Autodesk Inventor part; units mm, degrees
(part 9 of 18)
  spline S29 degree 3 poles (-103.2775, -7.9462) (-103.2327, -7.9264) (-103.1438, -7.8872) (-103.011, -7.831) (-102.8802, -7.7775) (-102.7099, -7.7106) (-102.5013, -7.6329) (-102.3337, -7.5779) (-102.2514, -7.5508) knots 0 0 0 0 0.13379 0.264806 0.393183 0.519054 0.763783 1 1 1 1
  line L388 (-103.3326, -8.4726) -> (-103.2775, -7.9462)
  spline S30 degree 3 poles (-104.4053, -7.5885) (-104.4187, -7.5896) (-104.4452, -7.5917) (-104.4843, -7.5938) (-104.5221, -7.5949) (-104.5584, -7.595) (-104.5931, -7.594) (-104.6258, -7.5919) (-104.6567, -7.5887) (-104.6856, -7.5845) (-104.7125, -7.5794) (-104.7374, -7.5733) (-104.7601, -7.5664) (-104.7808, -7.5587) (-104.7995, -7.5501) (-104.8165, -7.5405) (-104.8319, -7.5301) (-104.8411, -7.5221) (-104.8455, -7.5181) knots 0 0 0 0 0.088475 0.174424 0.25743 0.337089 0.413015 0.484966 0.552919 0.616878 0.676853 0.732867 0.784956 0.833184 0.87778 0.920162 0.960829 1 1 1 1
  ellipse E254 centre (-100.1455, -8.2742) end of major axis (-105.5768, -7.7059) minor radius 0.0004 (-103.2775, -7.9462) -> (-105.5768, -7.7059) ccw
  line L389 (-105.263, -7.4516) -> (-105.5768, -7.7059)
  line L390 (-105.635, -8.2625) -> (-105.5768, -7.7059)
  spline S31 degree 3 poles (-100.1515, -7.8096) (-100.1089, -7.7854) (-100.0246, -7.7374) (-99.8983, -7.6681) (-99.7738, -7.6016) (-99.6114, -7.5178) (-99.412, -7.4194) (-99.2511, -7.3476) (-99.172, -7.3123) knots 0 0 0 0 0.133763 0.26476 0.393126 0.518994 0.763738 1 1 1 1
  line L391 (-100.1515, -7.9913) -> (-100.1515, -7.8096)
  line L392 (-93.8516, -7.8096) -> (-93.8516, -7.9913)
  spline S32 degree 3 poles (-94.8311, -7.3123) (-94.752, -7.3476) (-94.5911, -7.4194) (-94.3917, -7.5178) (-94.2292, -7.6016) (-94.1047, -7.6681) (-93.9785, -7.7374) (-93.8942, -7.7854) (-93.8516, -7.8096) knots 0 0 0 0 0.236262 0.481006 0.606874 0.73524 0.866237 1 1 1 1
  line L393 (-99.172, -7.3123) -> (-94.8311, -7.3123)
  ellipse E255 centre (-97.0015, -7.7766) end of major axis (-101.9625, -7.7766) minor radius 0.5163 (-94.327, -7.3418) -> (-94.8311, -7.3123) ccw
  ellipse E256 centre (-97.0015, -7.7766) end of major axis (-101.9625, -7.7766) minor radius 0.5163 (-99.172, -7.3123) -> (-99.6761, -7.3418) ccw
  ellipse E257 centre (-97.0015, -8.2739) end of major axis (-91.5405, -8.2739) minor radius 0.5683 (-91.7042, -8.1358) -> (-93.8516, -7.8096) ccw
  ellipse E258 centre (-97.0015, -8.2739) end of major axis (-102.4625, -8.2739) minor radius 0.5683 (-100.1515, -7.8096) -> (-102.2989, -8.1358) ccw
  line L394 (-90.7255, -7.9462) -> (-90.6705, -8.4726)
  spline S33 degree 3 poles (-91.7517, -7.5508) (-91.6694, -7.5779) (-91.5018, -7.6329) (-91.2932, -7.7106) (-91.1229, -7.7775) (-90.9921, -7.831) (-90.8593, -7.8872) (-90.7704, -7.9264) (-90.7255, -7.9462) knots 0 0 0 0 0.236217 0.480946 0.606817 0.735194 0.86621 1 1 1 1
  spline S34 degree 3 poles (-89.158, -7.5179) (-89.1627, -7.5219) (-89.1722, -7.5302) (-89.1885, -7.5409) (-89.2064, -7.5508) (-89.2261, -7.5597) (-89.2476, -7.5676) (-89.2708, -7.5745) (-89.2958, -7.5805) (-89.3224, -7.5854) (-89.3508, -7.5893) (-89.381, -7.5922) (-89.413, -7.5941) (-89.4468, -7.5949) (-89.4823, -7.5947) (-89.5195, -7.5936) (-89.5583, -7.5915) (-89.5847, -7.5893) (-89.5982, -7.5882) knots 0 0 0 0 0.040391 0.082789 0.1275 0.174786 0.22486 0.277901 0.334055 0.393442 0.45616 0.522411 0.592561 0.666584 0.744418 0.825989 0.911213 1 1 1 1
  ellipse E259 centre (-93.8576, -8.2742) end of major axis (-88.4263, -7.7059) minor radius 0.0004 (-88.4263, -7.7059) -> (-90.7255, -7.9462) ccw
  line L395 (-88.7401, -7.4516) -> (-88.4263, -7.7059)
  line L396 (-88.368, -8.2625) -> (-88.4263, -7.7059)
  spline S35 degree 3 poles (-102.8055, -6.0195) (-102.7608, -5.9992) (-102.6724, -5.9592) (-102.5401, -5.9017) (-102.4098, -5.8469) (-102.2402, -5.7784) (-102.0323, -5.6987) (-101.8653, -5.642) (-101.7833, -5.6141) knots 0 0 0 0 0.13379 0.264806 0.393183 0.519054 0.763783 1 1 1 1
  line L397 (-102.9759, -7.8167) -> (-102.8055, -6.0195)
  line L398 (-101.7833, -5.6141) -> (-100.9875, -5.6895)
  ellipse E260 centre (-99.6228, -5.819) end of major axis (-104.5617, -5.3508) minor radius 0.0001 (-104.3919, -5.3669) -> (-104.5617, -5.3508) ccw
  ellipse E261 centre (-99.6228, -5.819) end of major axis (-104.5617, -5.3508) minor radius 0.0001 (-101.7833, -5.6141) -> (-103.1187, -5.4876) ccw
  spline S36 degree 3 poles (-103.1187, -5.4876) (-103.1703, -5.5034) (-103.2713, -5.5344) (-103.4207, -5.5753) (-103.5636, -5.6103) (-103.6994, -5.6388) (-103.8283, -5.6607) (-103.9499, -5.6751) (-104.0464, -5.6809) (-104.118, -5.6805) (-104.1663, -5.6778) (-104.2103, -5.6727) (-104.2501, -5.6655) (-104.2854, -5.6563) (-104.3249, -5.6422) (-104.3662, -5.6193) (-104.4034, -5.5814) (-104.4244, -5.5341) (-104.4269, -5.4805) (-104.4157, -5.4236) (-104.4001, -5.3864) (-104.3919, -5.3669) knots 0 0 0 0 0.104135 0.203976 0.298889 0.388275 0.471711 0.551067 0.624597 0.658204 0.689291 0.717816 0.743784 0.767218 0.788166 0.824633 0.857384 0.888881 0.922221 0.959245 1 1 1 1
  ellipse E262 centre (-99.67, -6.3167) end of major axis (-105.1066, -5.8014) minor radius 0.0001 (-102.8056, -6.0195) -> (-105.1066, -5.8014) ccw
  line L399 (-104.5617, -5.3508) -> (-105.1066, -5.8014)
  ellipse E263 centre (-103.0608, -5.4931) end of major axis (-101.5562, -5.6357) minor radius 0 (-104.3923, -5.3669) -> (-103.2014, -5.4797) ccw
  line L400 (-105.263, -7.4516) -> (-105.1066, -5.8014)
  spline S37 degree 3 poles (-100.1515, -5.896) (-100.1089, -5.8717) (-100.0246, -5.8237) (-99.8983, -5.7543) (-99.7738, -5.6878) (-99.6114, -5.6039) (-99.412, -5.5054) (-99.2511, -5.4335) (-99.172, -5.3982) knots 0 0 0 0 0.133768 0.264768 0.393136 0.519004 0.763746 1 1 1 1
  line L401 (-100.1515, -7.6101) -> (-100.1515, -5.896)
  line L402 (-93.8516, -5.896) -> (-93.8516, -7.6101)
  spline S38 degree 3 poles (-94.8311, -5.3982) (-94.752, -5.4335) (-94.5911, -5.5054) (-94.3917, -5.6039) (-94.2292, -5.6878) (-94.1047, -5.7543) (-93.9785, -5.8237) (-93.8942, -5.8717) (-93.8516, -5.896) knots 0 0 0 0 0.236254 0.480996 0.606864 0.735232 0.866232 1 1 1 1
  line L403 (-99.172, -5.3982) -> (-94.8311, -5.3982)
  ellipse E264 centre (-97.0015, -5.819) end of major axis (-101.9625, -5.819) minor radius 0.4679 (-93.4897, -5.4885) -> (-94.8311, -5.3982) ccw
  ellipse E265 centre (-97.0015, -5.819) end of major axis (-101.9625, -5.819) minor radius 0.4679 (-99.172, -5.3982) -> (-100.5134, -5.4885) ccw
  spline S39 degree 3 poles (-100.5134, -5.4885) (-100.5535, -5.5066) (-100.6325, -5.5425) (-100.7498, -5.5934) (-100.8637, -5.6409) (-100.9737, -5.6846) (-101.0793, -5.7244) (-101.1807, -5.7602) (-101.2782, -5.7918) (-101.3715, -5.8191) (-101.4585, -5.8412) (-101.5371, -5.8571) (-101.6059, -5.8666) (-101.664, -5.8701) (-101.7122, -5.8679) (-101.7509, -5.8595) (-101.7824, -5.8458) (-101.796, -5.8302) (-101.8023, -5.823) knots 0 0 0 0 0.096483 0.190064 0.280343 0.366935 0.449463 0.527566 0.602572 0.674179 0.740358 0.79923 0.84998 0.89243 0.926709 0.955226 0.979191 1 1 1 1
  spline S40 degree 3 poles (-92.2008, -5.823) (-92.207, -5.8301) (-92.2203, -5.8454) (-92.2514, -5.8588) (-92.2901, -5.8672) (-92.3377, -5.8698) (-92.3937, -5.8669) (-92.4583, -5.8584) (-92.5314, -5.8439) (-92.6132, -5.8239) (-92.7029, -5.7983) (-92.8, -5.7675) (-92.9036, -5.7316) (-93.0131, -5.6909) (-93.1275, -5.6457) (-93.2876, -5.5793) (-93.4082, -5.5251) (-93.4897, -5.4885) knots 0 0 0 0 0.020314 0.043937 0.072556 0.107061 0.147904 0.195304 0.249736 0.311344 0.379674 0.454238 0.534533 0.62004 0.710199 0.804177 1 1 1 1
  ellipse E266 centre (-97.0015, -6.3168) end of major axis (-91.5405, -6.3168) minor radius 0.5151 (-91.8465, -6.1468) -> (-93.8516, -5.896) ccw
  ellipse E267 centre (-97.0015, -6.3168) end of major axis (-102.4625, -6.3168) minor radius 0.5151 (-100.1515, -5.896) -> (-102.1566, -6.1468) ccw
  line L404 (-91.1976, -6.0195) -> (-91.0272, -7.8167)
  spline S41 degree 3 poles (-92.2198, -5.6141) (-92.1378, -5.642) (-91.9707, -5.6987) (-91.7629, -5.7784) (-91.5932, -5.8469) (-91.463, -5.9017) (-91.3307, -5.9592) (-91.2423, -5.9992) (-91.1976, -6.0195) knots 0 0 0 0 0.236217 0.480946 0.606817 0.735194 0.86621 1 1 1 1
  line L405 (-93.0155, -5.6895) -> (-92.2198, -5.6141)
  ellipse E268 centre (-94.3803, -5.819) end of major axis (-99.3192, -6.2871) minor radius 0.0001 (-90.8829, -5.4874) -> (-92.218, -5.6139) ccw
  ellipse E269 centre (-94.3803, -5.819) end of major axis (-89.4414, -5.3508) minor radius 0.0001 (-89.4414, -5.3508) -> (-89.6112, -5.3669) ccw
  spline S42 degree 3 poles (-89.6112, -5.3669) (-89.6028, -5.3869) (-89.5869, -5.4245) (-89.576, -5.4815) (-89.5789, -5.534) (-89.5992, -5.5805) (-89.6362, -5.6181) (-89.6877, -5.6467) (-89.7531, -5.6669) (-89.8324, -5.6786) (-89.9257, -5.6817) (-90.0326, -5.6767) (-90.1522, -5.6636) (-90.2831, -5.6426) (-90.4238, -5.614) (-90.5724, -5.5779) (-90.7271, -5.5358) (-90.8314, -5.5038) (-90.8844, -5.4876) knots 0 0 0 0 0.041849 0.07857 0.111147 0.141904 0.174268 0.211184 0.254599 0.305659 0.365519 0.434561 0.512207 0.59776 0.690456 0.789354 0.89303 1 1 1 1
  ellipse E270 centre (-94.3331, -6.3167) end of major axis (-88.8965, -5.8014) minor radius 0.0001 (-88.8965, -5.8014) -> (-91.1976, -6.0195) ccw
  line L406 (-89.4414, -5.3508) -> (-88.8965, -5.8014)
  line L407 (-88.7401, -7.4516) -> (-88.8965, -5.8014)
  ellipse E271 centre (-99.8333, -5.2905) end of major axis (-103.727, -4.8831) minor radius 0.0003 (-100.193, -5.2526) -> (-101.4573, -5.1203) ccw
  ellipse E272 centre (-101.7722, -5.0874) end of major axis (-101.5733, -5.1082) minor radius 0 (-101.6634, -5.0988) -> (-101.5733, -5.1082) ccw
  line L408 (-101.5732, -5.1082) -> (-101.5733, -5.1082)
  ellipse E273 centre (-101.3743, -5.129) end of major axis (-101.5732, -5.1082) minor radius 0 (-101.4573, -5.1203) -> (-101.5732, -5.1082) ccw
  ellipse E274 centre (-99.8333, -5.2905) end of major axis (-103.18, -4.9403) minor radius 0.0002 (-101.6634, -5.0988) -> (-103.18, -4.9403) ccw
  line L409 (-103.18, -4.9403) -> (-103.2361, -5.4765)
  ellipse E275 centre (-98.1892, 10.4238) end of major axis (-100.4369, 10.6589) minor radius 0.0002 (-100.1627, 10.6303) -> (-100.4369, 10.6589) ccw
  line L410 (-100.4369, 10.6589) -> (-100.7333, 8.7118)
  line L411 (-95.2515, -5.3982) -> (-95.2515, -4.9388)
  ellipse E276 centre (-95.4515, -4.9388) end of major axis (-95.2515, -4.9388) minor radius 0.0208 (-95.2515, -4.9388) -> (-95.3681, -4.9199) ccw
  ellipse E277 centre (-97.0015, -5.2902) end of major axis (-100.9165, -5.2902) minor radius 0.4074 (-95.3681, -4.9199) -> (-98.635, -4.9199) ccw
  ellipse E278 centre (-95.0515, -4.9796) end of major axis (-95.2515, -4.9796) minor radius 0.0208 (-95.2515, -4.9796) -> (-95.1609, -4.997) ccw
  ellipse E279 centre (-98.9515, -4.9796) end of major axis (-98.7515, -4.9796) minor radius 0.0208 (-98.8421, -4.997) -> (-98.7515, -4.9796) ccw
  ellipse E280 centre (-98.5515, -4.9388) end of major axis (-98.7515, -4.9388) minor radius 0.0208 (-98.635, -4.9199) -> (-98.7515, -4.9388) ccw
  line L412 (-98.7515, -4.9388) -> (-98.7515, -5.3982)
  ellipse E281 centre (-97.0015, -5.2902) end of major axis (-93.6365, -5.2902) minor radius 0.3502 (-93.6737, -5.2383) -> (-95.1609, -4.997) ccw
  ellipse E282 centre (-97.0015, -5.2902) end of major axis (-100.3665, -5.2902) minor radius 0.3502 (-98.8421, -4.997) -> (-100.3294, -5.2383) ccw
  ellipse E283 centre (-97.0015, 10.424) end of major axis (-94.7415, 10.424) minor radius 0.2352 (-95.9635, 10.6329) -> (-98.0396, 10.6329) ccw
  ellipse E284 centre (-92.6288, -5.129) end of major axis (-92.4299, -5.1082) minor radius 0 (-92.4299, -5.1082) -> (-92.5458, -5.1203) ccw
  ellipse E285 centre (-94.1698, -5.2905) end of major axis (-98.0636, -5.6979) minor radius 0.0003 (-92.5458, -5.1203) -> (-93.8101, -5.2526) ccw
  line L413 (-92.4298, -5.1082) -> (-92.4299, -5.1082)
  ellipse E286 centre (-92.2309, -5.0874) end of major axis (-92.4298, -5.1082) minor radius 0 (-92.4298, -5.1082) -> (-92.3397, -5.0988) ccw
  ellipse E287 centre (-94.1698, -5.2905) end of major axis (-90.8231, -4.9403) minor radius 0.0002 (-90.8231, -4.9403) -> (-92.3397, -5.0988) ccw
  line L414 (-90.8231, -4.9403) -> (-90.767, -5.4765)
  ellipse E288 centre (-95.8139, 10.4238) end of major axis (-93.5662, 10.6589) minor radius 0.0002 (-93.5662, 10.6589) -> (-93.8403, 10.6303) ccw
  line L415 (-93.5662, 10.6589) -> (-93.2698, 8.7118)
  ellipse E289 centre (-98.5408, 8.4556) end of major axis (-100.7855, 8.7179) minor radius 0.0001 (-100.0274, 8.6294) -> (-100.7855, 8.7179) ccw
  line L416 (-100.7855, 8.7179) -> (-102.7163, -3.0145)
  line L417 (-102.7652, -3.3114) -> (-103.0357, -4.9553)
  ellipse E290 centre (-97.0015, -7.2372) end of major axis (-100.9165, -7.2372) minor radius 0.4538 (-96.2832, -6.7911) -> (-96.387, -6.789) ccw
  ellipse E291 centre (-97.0015, -7.2372) end of major axis (-100.9165, -7.2372) minor radius 0.4538 (-96.6609, -6.7851) -> (-97.3972, -6.7857) ccw
  ellipse E292 centre (-97.0015, -7.2372) end of major axis (-100.9165, -7.2372) minor radius 0.4538 (-97.6161, -6.789) -> (-97.7199, -6.7911) ccw
  ellipse E293 centre (-97.0015, 8.4563) end of major axis (-94.7415, 8.4563) minor radius 0.262 (-95.2926, 8.6277) -> (-98.7105, 8.6277) ccw
  ellipse E294 centre (-95.4623, 8.4556) end of major axis (-93.2176, 8.7179) minor radius 0.0001 (-93.2176, 8.7179) -> (-93.9757, 8.6294) ccw
  line L418 (-93.2176, 8.7179) -> (-91.2868, -3.0145)
  line L419 (-91.2379, -3.3114) -> (-90.9673, -4.9553)
  ellipse E295 centre (-97.8026, 13.3841) end of major axis (-97.5985, 13.3647) minor radius 0 (-97.5985, 13.3647) -> (-97.8444, 13.388) ccw
  ellipse E296 centre (-97.8437, 12.95) end of major axis (-99.0732, 13.0666) minor radius 0 (-98.1872, 12.9826) -> (-99.0732, 13.0666) ccw
  line L420 (-99.0732, 13.0666) -> (-99.1254, 12.5159)
  arc A2 (-98.1701, 13.3945) -> (-99.0732, 13.0666) centre (-97.9837, 11.4735) ccw
  arc A3 (-97.4927, 13.34) -> (-97.5985, 13.3647) centre (-97.9837, 11.4735) ccw
  ellipse E297 centre (-99.3869, -3.3301) end of major axis (-103.2844, -2.9607) minor radius 0 (-100.0249, -3.2696) -> (-101.0128, -3.176) ccw
  ellipse E298 centre (-99.4812, -4.3257) end of major axis (-103.3788, -3.9562) minor radius 0 (-99.7317, -4.3019) -> (-101.1071, -4.1715) ccw
  line L421 (-101.1288, -3.165) -> (-101.1289, -3.165)
  line L422 (-101.2232, -4.1605) -> (-101.2232, -4.1605)
  ellipse E299 centre (-99.3869, -3.3301) end of major axis (-102.7369, -3.0126) minor radius 0 (-101.2191, -3.1564) -> (-102.7369, -3.0126) ccw
  ellipse E300 centre (-99.4812, -4.3257) end of major axis (-102.8312, -4.0081) minor radius 0 (-101.3134, -4.152) -> (-102.59, -4.031) ccw
  line L423 (-102.7369, -3.0126) -> (-102.7652, -3.3114)
  ellipse E301 centre (-97.8959, 12.3994) end of major axis (-100.1459, 12.6126) minor radius 0 (-98.9808, 12.5022) -> (-100.1459, 12.6126) ccw
  line L424 (-100.1459, 12.6126) -> (-100.424, 10.6576)
  ellipse E302 centre (-97.0015, 12.9501) end of major axis (-95.7665, 12.9501) minor radius 0.1165 (-95.8159, 12.9827) -> (-98.1872, 12.9827) ccw
  arc A4 (-97.2057, 13.3927) -> (-97.9832, 13.1353) centre (-97.0015, 11.4736) ccw
  arc A5 (-96.0199, 13.1353) -> (-96.7974, 13.3927) centre (-97.0015, 11.4736) ccw
  ellipse E303 centre (-95.4515, -4.0072) end of major axis (-95.2515, -4.0072) minor radius 0.0189 (-95.2515, -4.0072) -> (-95.3681, -3.9901) ccw
  line L425 (-95.2515, -4.0072) -> (-95.2515, -3.0117)
  ellipse E304 centre (-95.4515, -3.0117) end of major axis (-95.2515, -3.0117) minor radius 0.0189 (-95.2515, -3.0117) -> (-95.3681, -2.9945) ccw
  ellipse E305 centre (-97.0015, -3.3301) end of major axis (-100.9165, -3.3301) minor radius 0.3693 (-95.3681, -2.9945) -> (-98.635, -2.9945) ccw
  ellipse E306 centre (-97.0015, -4.3257) end of major axis (-100.9165, -4.3257) minor radius 0.3693 (-95.3681, -3.9901) -> (-98.635, -3.9901) ccw
  ellipse E307 centre (-95.0515, -3.0486) end of major axis (-95.2515, -3.0486) minor radius 0.0189 (-95.2515, -3.0486) -> (-95.1609, -3.0644) ccw
  ellipse E308 centre (-98.9515, -3.0486) end of major axis (-98.7515, -3.0486) minor radius 0.0189 (-98.8421, -3.0644) -> (-98.7515, -3.0486) ccw
  ellipse E309 centre (-98.5515, -3.0117) end of major axis (-98.7515, -3.0117) minor radius 0.0189 (-98.635, -2.9945) -> (-98.7515, -3.0117) ccw
  ellipse E310 centre (-98.5515, -4.0072) end of major axis (-98.7515, -4.0072) minor radius 0.0189 (-98.635, -3.9901) -> (-98.7515, -4.0072) ccw
  line L426 (-98.7515, -3.0117) -> (-98.7515, -4.0072)
  ellipse E311 centre (-95.0515, -4.0442) end of major axis (-95.2515, -4.0442) minor radius 0.0189 (-95.2515, -4.0442) -> (-95.1609, -4.06) ccw
  line L427 (-95.2515, -4.0442) -> (-95.2515, -4.0072)
  ellipse E312 centre (-98.9515, -4.0442) end of major axis (-98.7515, -4.0442) minor radius 0.0189 (-98.8421, -4.06) -> (-98.7515, -4.0442) ccw
  line L428 (-98.7515, -4.0072) -> (-98.7515, -4.0442)
  ellipse E313 centre (-97.0015, -3.3301) end of major axis (-93.6365, -3.3301) minor radius 0.3174 (-93.751, -3.2481) -> (-95.1609, -3.0644) ccw
  ellipse E314 centre (-97.0015, -3.3301) end of major axis (-100.3665, -3.3301) minor radius 0.3174 (-98.8421, -3.0644) -> (-100.2521, -3.2481) ccw
  ellipse E315 centre (-97.0015, -4.3257) end of major axis (-100.3665, -4.3257) minor radius 0.3174 (-100.2714, -4.2507) -> (-100.3408, -4.2865) ccw
  ellipse E316 centre (-97.0015, -4.3257) end of major axis (-93.6365, -4.3257) minor radius 0.3174 (-98.8421, -4.06) -> (-100.0624, -4.1938) ccw
  ellipse E317 centre (-97.0015, -4.3257) end of major axis (-93.6365, -4.3257) minor radius 0.3174 (-93.9407, -4.1938) -> (-95.1609, -4.06) ccw
  ellipse E318 centre (-97.0015, -4.3257) end of major axis (-93.6365, -4.3257) minor radius 0.3174 (-93.6623, -4.2865) -> (-93.7317, -4.2507) ccw
  ellipse E319 centre (-97.0015, 12.3994) end of major axis (-94.7415, 12.3994) minor radius 0.2132 (-95.0219, 12.5023) -> (-98.9812, 12.5023) ccw
  ellipse E320 centre (-96.2005, 13.3841) end of major axis (-96.4046, 13.3647) minor radius 0 (-96.1587, 13.388) -> (-96.4046, 13.3647) ccw
  ellipse E321 centre (-96.1593, 12.95) end of major axis (-94.9298, 13.0666) minor radius 0 (-94.9298, 13.0666) -> (-95.8159, 12.9826) ccw
  line L429 (-94.9298, 13.0666) -> (-94.8777, 12.5159)
  arc A6 (-96.4046, 13.3647) -> (-96.5104, 13.34) centre (-96.0194, 11.4735) ccw
  arc A7 (-94.9298, 13.0666) -> (-95.833, 13.3945) centre (-96.0194, 11.4735) ccw
  ellipse E322 centre (-94.6162, -3.3301) end of major axis (-98.5137, -3.6995) minor radius 0 (-92.9898, -3.1759) -> (-93.9776, -3.2695) ccw
  ellipse E323 centre (-94.5218, -4.3257) end of major axis (-98.4194, -4.6951) minor radius 0 (-92.8954, -4.1715) -> (-94.2709, -4.3018) ccw
  line L430 (-92.8742, -3.165) -> (-92.8743, -3.165)
  line L431 (-92.7799, -4.1605) -> (-92.7799, -4.1605)
  ellipse E324 centre (-94.6162, -3.3301) end of major axis (-91.2662, -3.0126) minor radius 0 (-91.2662, -3.0126) -> (-92.7841, -3.1564) ccw
  ellipse E325 centre (-94.5218, -4.3257) end of major axis (-91.1719, -4.0081) minor radius 0 (-91.4131, -4.031) -> (-92.6897, -4.152) ccw
  line L432 (-91.2662, -3.0126) -> (-91.2379, -3.3114)
  ellipse E326 centre (-96.1071, 12.3994) end of major axis (-93.8572, 12.6126) minor radius 0 (-93.8572, 12.6126) -> (-95.0222, 12.5022) ccw
  line L433 (-93.8572, 12.6126) -> (-93.5791, 10.6576)
  line L434 (-89.8363, -39.8016) -> (-90.502, -38.0864)
  line L435 (-87.7616, -39.8016) -> (-88.3038, -37.921)
  line L436 (-106.7956, -39.8016) -> (-106.8977, -37.7823)
  line L437 (-104.7253, -39.8016) -> (-104.6228, -37.8506)
  line L438 (-89.8808, -39.139) -> (-90.114, -38.0389)
  line L439 (-87.7498, -39.0854) -> (-87.8913, -37.8305)
  line L440 (-106.2533, -39.0854) -> (-106.1118, -37.8305)
  line L441 (-104.1223, -39.139) -> (-103.8891, -38.0389)
  line L442 (-89.2778, -39.8016) -> (-89.3803, -37.8506)
  line L443 (-87.2075, -39.8016) -> (-87.1064, -37.8014)
  line L444 (-106.2415, -39.8016) -> (-105.697, -37.9132)
  line L445 (-104.1668, -39.8016) -> (-103.5011, -38.0864)
  line L446 (-89.6018, -38.3908) -> (-89.6845, -37.9452)
  line L447 (-87.4159, -38.4054) -> (-87.4766, -37.7841)
  line L448 (-106.5872, -38.4054) -> (-106.5265, -37.7841)
  line L449 (-104.4013, -38.3908) -> (-104.3186, -37.9452)
  ellipse E327 centre (-107.4245, -24.551) end of major axis (-107.4978, -24.3758) minor radius 0.1721 (-107.5993, -24.5429) -> (-107.4934, -24.7177) ccw
  ellipse E328 centre (-107.4831, -24.5756) end of major axis (-107.4098, -24.7509) minor radius 0.1721 (-107.6185, -24.6838) -> (-107.5602, -24.7376) ccw
  ellipse E329 centre (-107.4131, -27.3549) end of major axis (-107.4865, -27.1797) minor radius 0.1721 (-107.5253, -27.2031) -> (-107.5455, -27.2228) ccw
  ellipse E330 centre (-107.6745, -24.5739) end of major axis (-107.6834, -24.7637) minor radius 0.074 (-107.6698, -24.7612) -> (-107.6002, -24.5428) ccw
  ellipse E331 centre (-107.8125, -24.5675) end of major axis (-107.8214, -24.7573) minor radius 0.074 (-107.8078, -24.7547) -> (-107.7382, -24.5364) ccw
  ellipse E332 centre (-107.7425, -27.3468) end of major axis (-107.7336, -27.157) minor radius 0.074 (-107.6682, -27.3157) -> (-107.7472, -27.1595) ccw
  ellipse E333 centre (-107.3545, -27.3304) end of major axis (-107.4278, -27.1551) minor radius 0.1721 (-107.4586, -27.1723) -> (-107.5293, -27.3222) ccw
  ellipse E334 centre (-107.6045, -27.3533) end of major axis (-107.5956, -27.1635) minor radius 0.074 (-107.5302, -27.3222) -> (-107.5956, -27.1635) ccw
  line L450 (-107.5956, -27.1635) -> (-107.7336, -27.157)
  line L451 (-107.3205, -24.7702) -> (-107.4116, -24.766)
  line L452 (-107.3377, -24.7421) -> (-107.2188, -24.7477)
  line L453 (-106.7334, -27.0126) -> (-106.7444, -26.578)
  line L454 (-106.7796, -25.179) -> (-106.7846, -24.9823)
  line L455 (-108.0455, -24.8542) -> (-107.8078, -24.7547)
  line L456 (-107.6698, -24.7612) -> (-107.8004, -24.8159)
  line L457 (-107.7472, -27.1595) -> (-107.8478, -27.2017)
  line L458 (-108.0687, -27.1049) -> (-108.1198, -25.0746)
  line L459 (-107.1516, -27.1528) -> (-107.233, -27.149)
  line L460 (-107.9818, -25.081) -> (-107.9307, -27.1113)
  line L461 (-106.7259, -24.9577) -> (-106.72, -25.1925)
  line L462 (-106.6941, -26.2206) -> (-106.6748, -26.988)
  ellipse E335 centre (-107.5179, -23.1958) end of major axis (-107.5913, -23.0205) minor radius 0.1721 (-107.5913, -23.0205) -> (-107.6503, -23.0636) ccw
  ellipse E336 centre (-107.3783, -28.7347) end of major axis (-107.305, -28.91) minor radius 0.1721 (-107.5137, -28.8429) -> (-107.5019, -28.8577) ccw
  ellipse E337 centre (-107.3197, -28.7102) end of major axis (-107.3931, -28.5349) minor radius 0.1721 (-107.4945, -28.702) -> (-107.435, -28.842) ccw
  ellipse E338 centre (-107.4592, -23.1712) end of major axis (-107.5326, -22.996) minor radius 0.1721 (-107.5178, -22.9906) -> (-107.6341, -23.1631) ccw
  line L463 (-107.5913, -23.0205) -> (-107.5326, -22.996)
  line L464 (-107.3519, -28.923) -> (-106.3387, -28.9703)
  line L465 (-107.4945, -28.702) -> (-107.5293, -27.3222)
  line L466 (-106.9273, -28.9155) -> (-107.2781, -28.8991)
  line L467 (-107.2501, -22.994) -> (-107.2016, -22.9962)
  line L468 (-107.5993, -24.5429) -> (-107.6341, -23.1631)
  ellipse E339 centre (-106.9082, -27.0044) end of major axis (-106.8349, -27.1797) minor radius 0.1721 (-106.7682, -27.127) -> (-106.7334, -27.0126) ccw
  ellipse E340 centre (-106.9594, -24.9741) end of major axis (-106.886, -25.1494) minor radius 0.1721 (-106.7846, -24.9823) -> (-106.7926, -24.9306) ccw
  ellipse E341 centre (-107.9944, -27.0738) end of major axis (-108.0032, -27.2636) minor radius 0.074 (-108.0687, -27.1049) -> (-108.0525, -27.2067) ccw
  ellipse E342 centre (-108.0455, -25.0435) end of major axis (-108.0367, -24.8537) minor radius 0.074 (-108.0631, -24.8645) -> (-108.1198, -25.0746) ccw
  ellipse E343 centre (-106.9007, -24.9496) end of major axis (-106.9741, -24.7743) minor radius 0.1721 (-106.7259, -24.9577) -> (-106.754, -24.859) ccw
  ellipse E344 centre (-106.8496, -26.9799) end of major axis (-106.7762, -27.1551) minor radius 0.1721 (-106.7344, -27.1293) -> (-106.6748, -26.988) ccw
  ellipse E345 centre (-107.8564, -27.0802) end of major axis (-107.8475, -26.8904) minor radius 0.074 (-107.9307, -27.1113) -> (-107.9206, -27.1924) ccw
  ellipse E346 centre (-107.9075, -25.0499) end of major axis (-107.8987, -24.8601) minor radius 0.074 (-107.9781, -25.0083) -> (-107.9818, -25.081) ccw
  line L469 (-107.7382, -24.5364) -> (-107.773, -23.1566)
  line L470 (-107.852, -23.0004) -> (-108.0369, -23.0778)
  line L471 (-108.1499, -29.1009) -> (-107.703, -28.9139)
  line L472 (-107.6334, -28.6955) -> (-107.6682, -27.3157)
  line L473 (-107.6002, -24.5428) -> (-107.635, -23.163)
  line L474 (-107.4954, -28.702) -> (-107.5302, -27.3222)
  line L475 (-108.4175, -29.2772) -> (-107.565, -28.9203)
  ellipse E347 centre (-107.8473, -23.1877) end of major axis (-107.8384, -22.9979) minor radius 0.074 (-107.773, -23.1566) -> (-107.852, -23.0004) ccw
  ellipse E348 centre (-107.7077, -28.7266) end of major axis (-107.7166, -28.9164) minor radius 0.074 (-107.703, -28.9139) -> (-107.6334, -28.6955) ccw
  ellipse E349 centre (-107.7093, -23.1941) end of major axis (-107.7004, -23.0043) minor radius 0.074 (-107.635, -23.163) -> (-107.7004, -23.0043) ccw
  ellipse E350 centre (-107.5697, -28.7331) end of major axis (-107.5786, -28.9229) minor radius 0.074 (-107.565, -28.9203) -> (-107.4954, -28.702) ccw
  line L476 (-107.8384, -22.9979) -> (-107.7004, -23.0043)
  line L477 (-107.649, -29.3585) -> (-108.2852, -29.3288)
  line L478 (-108.3439, -29.3534) -> (-107.6476, -29.3859)
  ellipse E351 centre (-108.1875, -29.2879) end of major axis (-108.4374, -29.2942) minor radius 0.0419 (-108.4175, -29.2772) -> (-108.2852, -29.3288) ccw
  ellipse E352 centre (-108.1875, -29.2879) end of major axis (-108.5873, -29.298) minor radius 0.067 (-108.5855, -29.2912) -> (-108.3439, -29.3534) ccw
  line L479 (-108.5875, -29.2921) -> (-108.5873, -29.298)
  line L480 (-87.5605, -24.7141) -> (-87.2796, -24.7036)
  line L481 (-87.4284, -26.9536) -> (-87.5613, -25.684)
  ellipse E353 centre (-87.3932, -23.1218) end of major axis (-87.4181, -22.9334) minor radius 0.1017 (-87.3138, -23.0264) -> (-87.413, -22.933) ccw
  line L482 (-87.413, -22.933) -> (-87.5162, -22.9368)
  line L483 (-87.3248, -28.9148) -> (-87.0301, -28.9039)
  line L484 (-87.0196, -28.9035) -> (-86.9511, -28.9009)
  line L485 (-87.5116, -28.9337) -> (-87.4053, -28.9298)
  ellipse E354 centre (-87.3264, -26.9498) end of major axis (-87.3015, -27.1381) minor radius 0.1017 (-87.4284, -26.9536) -> (-87.3388, -27.1307) ccw
  ellipse E355 centre (-87.5408, -24.9028) end of major axis (-87.5657, -24.7145) minor radius 0.1017 (-87.5605, -24.7141) -> (-87.5609, -24.7141) ccw
  line L486 (-106.3758, -22.9533) -> (-106.4658, -22.9531)
  line L487 (-106.7105, -28.9157) -> (-106.6709, -28.9157)
  line L488 (-106.4819, -28.916) -> (-106.2511, -28.9164)
  line L489 (-106.1582, -28.7277) -> (-106.0856, -28.0344)
  line L490 (-106.5872, -28.9325) -> (-106.5181, -28.9326)
  ellipse E356 centre (-106.2313, -28.7276) end of major axis (-106.2544, -28.9162) minor radius 0.0727 (-106.2511, -28.9164) -> (-106.1582, -28.7277) ccw
  line L491 (-106.22, -27.1474) -> (-106.2637, -27.1474)
  ellipse E357 centre (-106.0989, -22.9981) end of major axis (-106.4968, -22.9565) minor radius 0.0171 (-106.4658, -22.9531) -> (-106.4968, -22.9565) ccw
  line L492 (-106.4968, -22.9565) -> (-106.4973, -22.9614)
  line L493 (-85.5878, -29.276) -> (-85.977, -29.3087)
  line L494 (-86.3547, -29.3703) -> (-85.5063, -29.2991)
  ellipse E358 centre (-85.5831, -29.0888) end of major axis (-85.6349, -29.2716) minor radius 0.1568 (-85.5878, -29.276) -> (-85.5034, -29.2411) ccw
  ellipse E359 centre (-85.5016, -29.1118) end of major axis (-85.5534, -29.2946) minor radius 0.1568 (-85.5063, -29.2991) -> (-85.4195, -29.2623) ccw
  line L495 (-86.3274, -23.0058) -> (-86.3588, -22.9969)
  line L496 (-86.5078, -28.9104) -> (-86.068, -29.0349)
  line L497 (-86.5153, -28.9545) -> (-85.4493, -29.2564)
  line L498 (-86.403, -24.7513) -> (-86.0879, -24.8405)
  line L499 (-85.9894, -25.057) -> (-86.0405, -27.0873)
  ellipse E360 centre (-86.7386, -24.7794) end of major axis (-86.3388, -24.7895) minor radius 0.067 (-86.403, -24.7513) -> (-86.6279, -24.7178) ccw
  line L500 (-87.3612, -24.7519) -> (-87.0207, -24.7233)
  ellipse E361 centre (-86.7386, -24.7794) end of major axis (-86.9886, -24.7731) minor radius 0.0419 (-86.7545, -24.7373) -> (-86.8685, -24.7405) ccw
  line L501 (-86.3724, -24.8062) -> (-86.4378, -24.7876)
  ellipse E362 centre (-86.7992, -27.1842) end of major axis (-87.1991, -27.1742) minor radius 0.067 (-86.4734, -27.1534) -> (-86.7489, -27.119) ccw
  line L502 (-87.4582, -24.9769) -> (-87.4646, -25.2303)
  ellipse E363 centre (-86.0926, -25.0278) end of major axis (-86.1085, -24.8384) minor radius 0.1025 (-85.9894, -25.057) -> (-86.0879, -24.8405) ccw
  ellipse E364 centre (-86.1437, -27.0581) end of major axis (-86.1596, -26.8687) minor radius 0.1025 (-86.0684, -27.2021) -> (-86.0405, -27.0873) ccw
  ellipse E365 centre (-87.2988, -24.9635) end of major axis (-87.247, -24.7807) minor radius 0.1568 (-87.447, -24.9121) -> (-87.4582, -24.9769) ccw
  ellipse E366 centre (-87.3803, -24.9404) end of major axis (-87.432, -25.1232) minor radius 0.1568 (-87.4153, -24.7623) -> (-87.5126, -24.8518) ccw
  line L503 (-87.6665, -28.9578) -> (-87.3696, -28.9329)
  line L504 (-87.0376, -28.905) -> (-86.9793, -28.9001)
  ellipse E367 centre (-86.8434, -28.9386) end of major axis (-86.5935, -28.9449) minor radius 0.0419 (-86.8343, -28.897) -> (-86.9793, -28.9001) ccw
  ellipse E368 centre (-86.6944, -23.0251) end of major axis (-87.0943, -23.015) minor radius 0.067 (-86.3588, -22.9969) -> (-86.6623, -22.9591) ccw
  ellipse E369 centre (-86.8434, -28.9386) end of major axis (-87.2433, -28.9285) minor radius 0.067 (-86.5078, -28.9104) -> (-86.6724, -28.8822) ccw
  ellipse E370 centre (-85.4445, -29.0691) end of major axis (-85.4286, -29.2585) minor radius 0.1025 (-85.4493, -29.2564) -> (-85.4301, -29.2586) ccw
  line L505 (-87.9344, -29.3136) -> (-87.9787, -29.3011)
  ellipse E371 centre (-107.7625, -24.5841) end of major axis (-107.8385, -24.41) minor radius 0.169 (-107.9348, -24.5783) -> (-107.8445, -24.7402) ccw
  ellipse E372 centre (-107.8253, -24.6115) end of major axis (-107.7493, -24.7856) minor radius 0.169 (-107.9535, -24.7242) -> (-107.903, -24.7705) ccw
  ellipse E373 centre (-108.0152, -24.613) end of major axis (-108.0217, -24.8029) minor radius 0.0799 (-108.0058, -24.7997) -> (-107.9357, -24.5782) ccw
  ellipse E374 centre (-108.1512, -24.6084) end of major axis (-108.1577, -24.7983) minor radius 0.0799 (-108.1418, -24.7951) -> (-108.0717, -24.5736) ccw
  ellipse E375 centre (-108.0112, -27.3794) end of major axis (-108.0047, -27.1895) minor radius 0.0799 (-107.9316, -27.3447) -> (-108.0206, -27.1927) ccw
  ellipse E376 centre (-107.6224, -27.3551) end of major axis (-107.6984, -27.181) minor radius 0.169 (-107.7606, -27.2309) -> (-107.7947, -27.3493) ccw
  ellipse E377 centre (-107.8751, -27.384) end of major axis (-107.8687, -27.1941) minor radius 0.0799 (-107.7956, -27.3493) -> (-107.8687, -27.1941) ccw
  line L506 (-107.8687, -27.1941) -> (-108.0047, -27.1895)
  line L507 (-107.6857, -24.8026) -> (-107.7626, -24.8)
  line L508 (-107.6972, -24.7727) -> (-107.6219, -24.7752)
  line L509 (-107.025, -27.0322) -> (-107.0431, -26.6745)
  line L510 (-107.1176, -25.1998) -> (-107.1273, -25.0079)
  line L511 (-108.4015, -24.9085) -> (-108.1418, -24.7951)
  line L512 (-108.0058, -24.7997) -> (-108.2655, -24.9131)
  line L513 (-109.0549, -25.1939) -> (-108.812, -25.0878)
  line L514 (-108.723, -25.2397) -> (-108.6206, -27.264)
  line L515 (-108.6908, -27.4855) -> (-108.9337, -27.5916)
  line L516 (-108.0206, -27.1927) -> (-108.2803, -27.3062)
  line L517 (-108.3693, -27.1542) -> (-108.4716, -25.13)
  line L518 (-107.5467, -27.1713) -> (-107.5775, -27.1703)
  line L519 (-108.3356, -25.1346) -> (-108.2333, -27.1588)
  ellipse E378 centre (-108.6923, -25.2062) end of major axis (-109.0917, -25.2264) minor radius 0.0715 (-109.0549, -25.1939) -> (-108.8598, -25.2794) ccw
  line L520 (-108.7207, -25.2841) -> (-108.8598, -25.2794)
  line L521 (-108.797, -25.2519) -> (-108.7393, -25.2539)
  ellipse E379 centre (-108.6923, -25.2062) end of major axis (-108.9419, -25.2188) minor radius 0.0447 (-108.9189, -25.1985) -> (-108.797, -25.2519) ccw
  line L522 (-108.7494, -25.1245) -> (-108.9189, -25.1985)
  ellipse E380 centre (-108.571, -27.6038) end of major axis (-108.9705, -27.624) minor radius 0.0715 (-108.9337, -27.5916) -> (-108.9705, -27.624) ccw
  line L523 (-107.0645, -24.9805) -> (-107.0502, -25.2637)
  line L524 (-106.9799, -26.6541) -> (-106.9622, -27.0047)
  ellipse E381 centre (-107.8949, -23.2358) end of major axis (-107.9709, -23.0617) minor radius 0.169 (-107.9709, -23.0617) -> (-108.0251, -23.1016) ccw
  ellipse E382 centre (-107.6157, -28.7583) end of major axis (-107.5396, -28.9324) minor radius 0.169 (-107.6211, -28.9438) -> (-107.6062, -28.945) ccw
  ellipse E383 centre (-107.5528, -28.7308) end of major axis (-107.6289, -28.5567) minor radius 0.169 (-107.5578, -28.9164) -> (-107.5434, -28.9175) ccw
  ellipse E384 centre (-107.5528, -28.7308) end of major axis (-107.6289, -28.5567) minor radius 0.169 (-107.7251, -28.725) -> (-107.7079, -28.798) ccw
  ellipse E385 centre (-107.832, -23.2084) end of major axis (-107.9081, -23.0343) minor radius 0.169 (-107.902, -23.0318) -> (-108.0043, -23.2026) ccw
  line L525 (-107.9709, -23.0617) -> (-107.9081, -23.0343)
  line L526 (-107.6062, -28.945) -> (-107.5896, -28.9455)
  line L527 (-107.4377, -28.9507) -> (-106.3441, -28.9877)
  line L528 (-107.7251, -28.725) -> (-107.7947, -27.3493)
  line L529 (-107.2722, -28.9267) -> (-107.3548, -28.9239)
  line L530 (-107.5229, -28.9182) -> (-107.5434, -28.9175)
  line L531 (-107.6671, -23.0276) -> (-107.6493, -23.0282)
  line L532 (-107.9348, -24.5783) -> (-108.0043, -23.2026)
  ellipse E386 centre (-107.1973, -27.0263) end of major axis (-107.1212, -27.2004) minor radius 0.169 (-107.038, -27.1126) -> (-107.025, -27.0322) ccw
  ellipse E387 centre (-107.2996, -25.0021) end of major axis (-107.2235, -25.1762) minor radius 0.169 (-107.1273, -25.0079) -> (-107.1347, -24.9627) ccw
  ellipse E388 centre (-108.8025, -25.2745) end of major axis (-108.7961, -25.0846) minor radius 0.0799 (-108.723, -25.2397) -> (-108.812, -25.0878) ccw
  ellipse E389 centre (-108.7002, -27.2988) end of major axis (-108.7066, -27.4886) minor radius 0.0799 (-108.6908, -27.4855) -> (-108.6206, -27.264) ccw
  ellipse E390 centre (-108.2897, -27.1195) end of major axis (-108.2961, -27.3094) minor radius 0.0799 (-108.3693, -27.1542) -> (-108.2803, -27.3062) ccw
  ellipse E391 centre (-108.3921, -25.0952) end of major axis (-108.3856, -24.9053) minor radius 0.0799 (-108.4015, -24.9085) -> (-108.4716, -25.13) ccw
  ellipse E392 centre (-107.2368, -24.9746) end of major axis (-107.3128, -24.8005) minor radius 0.169 (-107.0645, -24.9805) -> (-107.0704, -24.9409) ccw
  ellipse E393 centre (-107.1344, -26.9989) end of major axis (-107.2105, -26.8248) minor radius 0.169 (-106.9966, -27.1236) -> (-106.9622, -27.0047) ccw
  ellipse E394 centre (-108.1537, -27.1241) end of major axis (-108.1473, -26.9342) minor radius 0.0799 (-108.2333, -27.1588) -> (-108.2069, -27.2741) ccw
  ellipse E395 centre (-108.2561, -25.0998) end of major axis (-108.2496, -24.9099) minor radius 0.0799 (-108.2655, -24.9131) -> (-108.3356, -25.1346) ccw
  line L533 (-108.0717, -24.5736) -> (-108.1412, -23.1979)
  line L534 (-108.2302, -23.046) -> (-109.1434, -23.4448)
  line L535 (-108.8453, -29.3407) -> (-107.9322, -28.9418)
  line L536 (-107.862, -28.7204) -> (-107.9316, -27.3447)
  line L537 (-107.9357, -24.5782) -> (-108.0052, -23.2025)
  line L538 (-107.726, -28.725) -> (-107.7956, -27.3493)
  line L539 (-108.7093, -29.3453) -> (-107.7962, -28.9464)
  ellipse E396 centre (-108.2208, -23.2327) end of major axis (-108.2144, -23.0428) minor radius 0.0799 (-108.1412, -23.1979) -> (-108.2302, -23.046) ccw
  ellipse E397 centre (-107.9416, -28.7551) end of major axis (-107.948, -28.945) minor radius 0.0799 (-107.9322, -28.9418) -> (-107.862, -28.7204) ccw
  ellipse E398 centre (-108.0848, -23.2373) end of major axis (-108.0784, -23.0474) minor radius 0.0799 (-108.0052, -23.2025) -> (-108.0784, -23.0474) ccw
  ellipse E399 centre (-107.8056, -28.7597) end of major axis (-107.812, -28.9496) minor radius 0.0799 (-107.7962, -28.9464) -> (-107.726, -28.725) ccw
  line L540 (-108.2144, -23.0428) -> (-108.0784, -23.0474)
  line L541 (-107.6453, -29.4306) -> (-108.5873, -29.3987)
  line L542 (-108.6501, -29.4261) -> (-107.6438, -29.4602)
  ellipse E400 centre (-108.4826, -29.3529) end of major axis (-108.7323, -29.3656) minor radius 0.0447 (-108.7093, -29.3453) -> (-108.5873, -29.3987) ccw
  ellipse E401 centre (-108.7807, -23.4571) end of major axis (-109.1802, -23.4773) minor radius 0.0715 (-109.1434, -23.4448) -> (-109.1802, -23.4773) ccw
  ellipse E402 centre (-108.4826, -29.3529) end of major axis (-108.8821, -29.3731) minor radius 0.0715 (-108.8453, -29.3407) -> (-108.6501, -29.4261) ccw
  line L543 (-109.1802, -23.4773) -> (-109.0917, -25.2264)
  line L544 (-108.9705, -27.624) -> (-108.8821, -29.3731)
  ellipse E403 centre (-87.3843, -24.4989) end of major axis (-87.3606, -24.6874) minor radius 0.0959 (-87.363, -24.6876) -> (-87.2885, -24.4916) ccw
  line L545 (-87.3606, -24.6874) -> (-87.3872, -24.6907)
  line L546 (-87.5622, -24.7028) -> (-87.363, -24.6876)
  line L547 (-87.206, -27.1206) -> (-87.402, -27.1355)
  line L548 (-87.519, -26.954) -> (-87.6192, -26.0659)
  line L549 (-87.2885, -24.4916) -> (-87.4454, -23.1007)
  line L550 (-87.5624, -22.9192) -> (-87.7687, -22.9349)
  line L551 (-87.9886, -28.9636) -> (-87.0478, -28.8921)
  line L552 (-88.0601, -28.9754) -> (-87.4292, -28.9274)
  ellipse E404 centre (-87.5411, -23.108) end of major axis (-87.5648, -22.9195) minor radius 0.0959 (-87.4454, -23.1007) -> (-87.5624, -22.9192) ccw
  ellipse E405 centre (-87.4233, -26.9467) end of major axis (-87.3996, -27.1352) minor radius 0.0959 (-87.519, -26.954) -> (-87.402, -27.1355) ccw
  ellipse E406 centre (-88.3312, -29.0066) end of major axis (-88.7287, -29.0514) minor radius 0.0085 (-87.9886, -28.9636) -> (-88.0593, -28.9697) ccw
  line L553 (-106.2348, -22.9385) -> (-106.3374, -22.9318)
  line L554 (-106.8615, -28.9024) -> (-106.1093, -28.9517)
  line L555 (-106.0096, -28.768) -> (-105.9946, -28.6348)
  line L556 (-106.5463, -28.9308) -> (-105.9738, -28.9683)
  line L557 (-106.5368, -24.7002) -> (-106.4413, -24.7065)
  line L558 (-106.3762, -26.1166) -> (-106.4709, -26.9564)
  line L559 (-106.5707, -27.14) -> (-106.8102, -27.1243)
  ellipse E407 centre (-106.1753, -24.7445) end of major axis (-106.5727, -24.6997) minor radius 0.0085 (-106.5368, -24.7002) -> (-106.5639, -24.6989) ccw
  ellipse E408 centre (-106.4486, -27.1686) end of major axis (-106.8461, -27.1238) minor radius 0.0085 (-106.8102, -27.1243) -> (-106.8461, -27.1238) ccw
  ellipse E409 centre (-106.5494, -26.9512) end of major axis (-106.5725, -27.1398) minor radius 0.0785 (-106.5707, -27.14) -> (-106.4709, -26.9564) ccw
  ellipse E410 centre (-106.0881, -28.7629) end of major axis (-106.1112, -28.9515) minor radius 0.0785 (-106.1093, -28.9517) -> (-106.0096, -28.768) ccw
  ellipse E411 centre (-105.9525, -28.7795) end of major axis (-105.9756, -28.9681) minor radius 0.0785 (-105.9738, -28.9683) -> (-105.9455, -28.9586) ccw
  ellipse E412 centre (-105.9758, -22.9761) end of major axis (-106.3733, -22.9313) minor radius 0.0085 (-106.3374, -22.9318) -> (-106.3733, -22.9313) ccw
  line L560 (-106.3733, -22.9313) -> (-106.3764, -22.9589)
  line L561 (-106.8461, -27.1238) -> (-106.8473, -27.1343)
  ellipse E413 centre (-85.031, -25.0552) end of major axis (-85.0938, -25.2345) minor radius 0.1599 (-85.0404, -25.2419) -> (-84.9429, -25.2009) ccw
  ellipse E414 centre (-85.1075, -25.0284) end of major axis (-85.1703, -25.2077) minor radius 0.1599 (-85.1169, -25.2151) -> (-85.0265, -25.1798) ccw
  ellipse E415 centre (-84.9639, -25.0118) end of major axis (-84.953, -25.2015) minor radius 0.0969 (-84.9733, -25.1985) -> (-84.953, -25.2015) ccw
  ellipse E416 centre (-84.8351, -25.0044) end of major axis (-84.8242, -25.1941) minor radius 0.0969 (-84.8445, -25.1911) -> (-84.7381, -25.0383) ccw
  ellipse E417 centre (-84.9752, -27.7754) end of major axis (-84.9861, -27.5857) minor radius 0.0969 (-84.8782, -27.8094) -> (-84.9657, -27.5887) ccw
  line L562 (-84.8242, -25.1941) -> (-84.953, -25.2015)
  line L563 (-85.2092, -25.2204) -> (-85.1169, -25.2151)
  line L564 (-85.0404, -25.2419) -> (-85.256, -25.2543)
  line L565 (-85.1607, -25.0802) -> (-84.8445, -25.1911)
  line L566 (-84.9733, -25.1985) -> (-85.2302, -25.1084)
  line L567 (-85.9564, -24.8013) -> (-85.6606, -24.905)
  line L568 (-85.5731, -25.1256) -> (-85.6754, -27.1499)
  line L569 (-85.7818, -27.3026) -> (-86.0776, -27.1989)
  line L570 (-84.9657, -27.5887) -> (-85.2819, -27.4779)
  line L571 (-85.3694, -27.2572) -> (-85.2671, -25.2329)
  ellipse E418 centre (-86.2999, -24.821) end of major axis (-85.9004, -24.8412) minor radius 0.0715 (-85.9564, -24.8013) -> (-86.3893, -24.7469) ccw
  ellipse E419 centre (-86.2999, -24.821) end of major axis (-86.5496, -24.8084) minor radius 0.0447 (-86.0852, -24.8087) -> (-86.2989, -24.7763) ccw
  line L572 (-85.7894, -24.9124) -> (-86.0852, -24.8087)
  ellipse E420 centre (-86.4211, -27.2186) end of major axis (-86.8206, -27.1984) minor radius 0.0715 (-86.0776, -27.1989) -> (-86.513, -27.1445) ccw
  line L573 (-85.8043, -27.1573) -> (-85.7019, -25.133)
  line L574 (-87.2056, -26.9434) -> (-87.1902, -26.6379)
  line L575 (-87.1285, -25.4188) -> (-87.1068, -24.9886)
  line L576 (-85.3266, -29.3618) -> (-86.3573, -29.4211)
  line L577 (-86.3589, -29.4524) -> (-85.25, -29.3886)
  ellipse E421 centre (-85.3171, -29.1751) end of major axis (-85.38, -29.3544) minor radius 0.1599 (-85.3266, -29.3618) -> (-85.2362, -29.3266) ccw
  ellipse E422 centre (-85.2406, -29.2019) end of major axis (-85.3035, -29.3812) minor radius 0.1599 (-85.25, -29.3886) -> (-85.1526, -29.3476) ccw
  line L578 (-84.7381, -25.0383) -> (-84.6686, -23.6626)
  line L579 (-84.7561, -23.442) -> (-85.868, -23.0521)
  line L580 (-86.1661, -28.948) -> (-85.0541, -29.3378)
  line L581 (-84.9478, -29.1851) -> (-84.8782, -27.8094)
  line L582 (-86.2949, -28.9554) -> (-85.1829, -29.3452)
  ellipse E423 centre (-84.7655, -23.6287) end of major axis (-84.7764, -23.439) minor radius 0.0969 (-84.6686, -23.6626) -> (-84.7561, -23.442) ccw
  ellipse E424 centre (-85.0447, -29.1511) end of major axis (-85.0338, -29.3408) minor radius 0.0969 (-85.0541, -29.3378) -> (-84.9478, -29.1851) ccw
  ellipse E425 centre (-85.1735, -29.1585) end of major axis (-85.1626, -29.3482) minor radius 0.0969 (-85.1829, -29.3452) -> (-85.1626, -29.3482) ccw
  line L583 (-85.0338, -29.3408) -> (-85.1626, -29.3482)
  ellipse E426 centre (-85.67, -25.0917) end of major axis (-85.6809, -24.902) minor radius 0.0969 (-85.5731, -25.1256) -> (-85.6606, -24.905) ccw
  ellipse E427 centre (-85.7724, -27.1159) end of major axis (-85.7615, -27.3056) minor radius 0.0969 (-85.7818, -27.3026) -> (-85.6754, -27.1499) ccw
  ellipse E428 centre (-85.2725, -27.2912) end of major axis (-85.2616, -27.4808) minor radius 0.0969 (-85.3694, -27.2572) -> (-85.2819, -27.4779) ccw
  ellipse E429 centre (-85.1702, -25.2669) end of major axis (-85.1811, -25.0772) minor radius 0.0969 (-85.1607, -25.0802) -> (-85.2671, -25.2329) ccw
  ellipse E430 centre (-85.7988, -25.0991) end of major axis (-85.8097, -24.9094) minor radius 0.0969 (-85.7019, -25.133) -> (-85.7894, -24.9124) ccw
  ellipse E431 centre (-86.8662, -24.9877) end of major axis (-86.8033, -24.8084) minor radius 0.1599 (-87.0256, -24.9663) -> (-87.0274, -24.9768) ccw
  ellipse E432 centre (-86.9427, -24.9609) end of major axis (-87.0056, -25.1402) minor radius 0.1599 (-87.1018, -24.9381) -> (-87.1043, -24.9533) ccw
  ellipse E433 centre (-87.045, -26.9851) end of major axis (-87.1079, -27.1644) minor radius 0.1599 (-87.2034, -27.0504) -> (-87.1733, -27.1161) ccw
  ellipse E434 centre (-86.9685, -27.0119) end of major axis (-86.9057, -26.8326) minor radius 0.1599 (-87.1293, -27.0654) -> (-87.1153, -27.1118) ccw
  ellipse E435 centre (-85.9012, -27.1233) end of major axis (-85.8903, -27.313) minor radius 0.0969 (-85.8411, -27.2818) -> (-85.8043, -27.1573) ccw
  line L584 (-87.3286, -28.9628) -> (-86.6995, -28.9266)
  line L585 (-86.8016, -28.9013) -> (-87.0021, -28.9128)
  line L586 (-87.3526, -28.933) -> (-87.4097, -28.9362)
  ellipse E436 centre (-86.5095, -28.9678) end of major axis (-86.2599, -28.9804) minor radius 0.0447 (-86.2949, -28.9554) -> (-86.4264, -28.9296) ccw
  ellipse E437 centre (-86.2115, -23.0719) end of major axis (-86.611, -23.0517) minor radius 0.0715 (-85.868, -23.0521) -> (-86.3548, -22.9981) ccw
  ellipse E438 centre (-86.5095, -28.9678) end of major axis (-86.909, -28.9476) minor radius 0.0715 (-86.1661, -28.948) -> (-86.5352, -28.8951) ccw
  ellipse E439 centre (-107.0376, -24.5247) end of major axis (-106.9792, -24.7055) minor radius 0.168 (-107.2077, -24.5125) -> (-107.0363, -24.7123) ccw
  ellipse E440 centre (-107.1043, -24.5462) end of major axis (-107.0459, -24.727) minor radius 0.168 (-107.2341, -24.6571) -> (-107.1031, -24.7338) ccw
  ellipse E441 centre (-107.0859, -27.3311) end of major axis (-107.1443, -27.1503) minor radius 0.168 (-107.1443, -27.1503) -> (-107.2078, -27.1904) ccw
  ellipse E442 centre (-107.2931, -24.5397) end of major axis (-107.3067, -24.7292) minor radius 0.0836 (-107.2919, -24.7273) -> (-107.2086, -24.5124) ccw
  ellipse E443 centre (-107.4275, -24.5301) end of major axis (-107.4411, -24.7196) minor radius 0.0836 (-107.4262, -24.7177) -> (-107.343, -24.5028) ccw
  ellipse E444 centre (-107.4091, -27.3149) end of major axis (-107.3955, -27.1254) minor radius 0.0836 (-107.3246, -27.2876) -> (-107.4104, -27.1273) ccw
  ellipse E445 centre (-107.0192, -27.3095) end of major axis (-107.0776, -27.1287) minor radius 0.168 (-107.0205, -27.1219) -> (-107.1894, -27.2973) ccw
  ellipse E446 centre (-107.2748, -27.3245) end of major axis (-107.2612, -27.135) minor radius 0.0836 (-107.1903, -27.2972) -> (-107.2612, -27.135) ccw
  line L587 (-107.0776, -27.1287) -> (-107.1443, -27.1503)
  line L588 (-107.2612, -27.135) -> (-107.3955, -27.1254)
  line L589 (-106.6024, -24.7697) -> (-107.1031, -24.7338)
  line L590 (-107.0363, -24.7123) -> (-106.5357, -24.7482)
  line L591 (-107.702, -24.8068) -> (-107.6889, -24.8025)
  line L592 (-107.6875, -24.8021) -> (-107.4262, -24.7177)
  line L593 (-107.2919, -24.7273) -> (-107.4621, -24.7823)
  line L594 (-107.4104, -27.1273) -> (-107.5645, -27.1771)
  line L595 (-107.7719, -27.056) -> (-107.7803, -25.7875)
  line L596 (-107.7832, -25.3462) -> (-107.7853, -25.0217)
  line L597 (-106.7634, -27.1403) -> (-107.0205, -27.1219)
  line L598 (-107.651, -25.0313) -> (-107.6493, -25.2877)
  line L599 (-107.6399, -26.7211) -> (-107.6376, -27.0657)
  ellipse E447 centre (-107.1134, -23.1637) end of major axis (-107.1718, -22.9829) minor radius 0.168 (-107.1718, -22.9829) -> (-107.2353, -23.023) ccw
  ellipse E448 centre (-107.0768, -28.7136) end of major axis (-107.0184, -28.8944) minor radius 0.168 (-107.2066, -28.8245) -> (-107.0756, -28.9012) ccw
  ellipse E449 centre (-107.0101, -28.6921) end of major axis (-106.9517, -28.8729) minor radius 0.168 (-107.1803, -28.6799) -> (-107.0089, -28.8797) ccw
  ellipse E450 centre (-107.0467, -23.1421) end of major axis (-107.1051, -22.9613) minor radius 0.168 (-107.0479, -22.9545) -> (-107.2168, -23.1299) ccw
  line L600 (-107.1718, -22.9829) -> (-107.1051, -22.9613)
  line L601 (-107.0756, -28.9012) -> (-106.8886, -28.9147)
  line L602 (-106.6278, -28.9333) -> (-106.2551, -28.9601)
  line L603 (-107.1803, -28.6799) -> (-107.1894, -27.2973)
  line L604 (-106.8321, -28.8924) -> (-107.0089, -28.8797)
  line L605 (-107.0479, -22.9545) -> (-106.6, -22.9866)
  line L606 (-107.2077, -24.5125) -> (-107.2168, -23.1299)
  ellipse E451 centre (-106.6012, -24.9574) end of major axis (-106.6596, -24.7766) minor radius 0.168 (-106.4598, -24.8643) -> (-106.6024, -24.7697) ccw
  ellipse E452 centre (-107.6874, -27.0287) end of major axis (-107.701, -27.2183) minor radius 0.0836 (-107.7719, -27.056) -> (-107.7601, -27.1459) ccw
  ellipse E453 centre (-107.7008, -24.9944) end of major axis (-107.6872, -24.8049) minor radius 0.0836 (-107.702, -24.8068) -> (-107.7166, -24.8143) ccw
  ellipse E454 centre (-107.7008, -24.9944) end of major axis (-107.7144, -25.1839) minor radius 0.0836 (-107.7788, -24.9447) -> (-107.7853, -25.0217) ccw
  ellipse E455 centre (-106.5345, -24.9358) end of major axis (-106.5929, -24.755) minor radius 0.168 (-106.4802, -24.7624) -> (-106.5357, -24.7482) ccw
  ellipse E456 centre (-107.5531, -27.0384) end of major axis (-107.5395, -26.8489) minor radius 0.0836 (-107.6376, -27.0657) -> (-107.6318, -27.1294) ccw
  ellipse E457 centre (-107.5665, -25.004) end of major axis (-107.5529, -24.8145) minor radius 0.0836 (-107.6445, -24.9542) -> (-107.651, -25.0313) ccw
  line L607 (-107.343, -24.5028) -> (-107.3521, -23.1202)
  line L608 (-107.4378, -22.9599) -> (-107.6636, -23.0328)
  line L609 (-107.7583, -29.0012) -> (-107.3988, -28.8851)
  line L610 (-107.3155, -28.6702) -> (-107.3246, -27.2876)
  line L611 (-107.2086, -24.5124) -> (-107.2177, -23.1298)
  line L612 (-107.1812, -28.6798) -> (-107.1903, -27.2972)
  line L613 (-108.2342, -29.208) -> (-107.2644, -28.8947)
  ellipse E458 centre (-107.4366, -23.1475) end of major axis (-107.423, -22.958) minor radius 0.0836 (-107.3521, -23.1202) -> (-107.4378, -22.9599) ccw